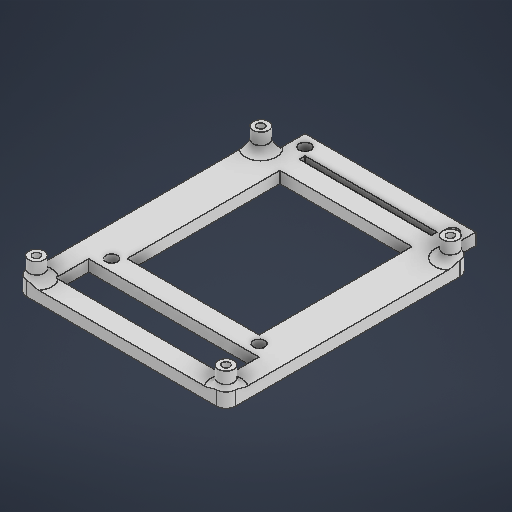
# Autodesk Inventor part: electronics_holder3
Saved by Autodesk Inventor 2026.1 (Build 301233000, 233)
## iProperties
Created: 2026-03-29
Part Number: electronics_holder3
Material: Generic
Document SubType Name: Modeling
Designer: emanuel
Density: 1 g/cm^3
Appearance: Default
Author: emanuel
Autodesk Inventor part; units mm, degrees
ref_plane "YZ Plane" through (0, 0, 0) normal (1, 0, 0) x (0, 1, 0)
ref_plane "XZ Plane" through (0, 0, 0) normal (0, 1, 0) x (-1, 0, 0)
ref_plane "XY Plane" through (0, 0, 0) normal (0, 0, 1) x (1, 0, 0)
sketch "Sketch1" plane through (0, 0, 0) normal (0, 1, 0) x (-1, 0, 0)
  line L0 (-19.075, 25) -> (19.075, 25)
  line L1 (19.075, 25) -> (19.075, -25)
  line L2 (19.075, -25) -> (-19.075, -25)
  line L3 (-19.075, -25) -> (-19.075, 25)
  line L4 (-19.075, 25) -> (19.075, -25) construction
  line L5 (19.075, 25) -> (-19.075, -25) construction
  circle A0 centre (19.075, 25) radius 1.5
  circle A1 centre (19.075, -25) radius 1.5
  circle A2 centre (-19.075, 25) radius 1.5
  circle A3 centre (-19.075, -25) radius 1.5
  line L6 (19.075, 25) -> (22.075, 25)
  line L7 (22.075, 25) -> (22.075, 28)
  line L8 (22.075, 28) -> (19.075, 28)
  line L9 (19.075, 28) -> (19.075, 25)
  line L10 (-19.075, -25) -> (-22.075, -25)
  line L11 (-22.075, -25) -> (-22.075, -28)
  line L12 (-22.075, -28) -> (-19.075, -28)
  line L13 (-19.075, -28) -> (-19.075, -25)
  line L14 (19.075, 25) -> (17.075, 25)
  line L15 (17.075, 25) -> (17.075, 23)
  line L16 (17.075, 23) -> (19.075, 23)
  line L17 (19.075, 23) -> (19.075, 25)
  line L18 (-19.075, -25) -> (-17.075, -25)
  line L19 (-17.075, -25) -> (-17.075, -23)
  line L20 (-17.075, -23) -> (-19.075, -23)
  line L21 (-19.075, -23) -> (-19.075, -25)
  line L22 (17.075, 23) -> (-17.075, 23)
  line L23 (-17.075, 23) -> (-17.075, -23)
  line L24 (-17.075, -23) -> (17.075, -23)
  line L25 (17.075, -23) -> (17.075, 23)
  line L26 (-22.075, -28) -> (22.075, -28)
  line L27 (22.075, -28) -> (22.075, 28)
  line L28 (22.075, 28) -> (-22.075, 28)
  line L29 (-22.075, 28) -> (-22.075, -28)
  point P0 (0, 0)
  dimension "d0" = 38.15
  dimension "d1" = 50
  dimension "d2" = 3
  dimension "d3" = 3
  dimension "d4" = 3
  dimension "d5" = 3
  dimension "d6" = 3
  dimension "d7" = 3
  dimension "d8" = 3
  dimension "d9" = 3
  dimension "d10" = 2
  dimension "d11" = 2
  dimension "d12" = 2
  dimension "d13" = 2
  constraints: 60 end point, 14 parallel, 7 horizontal, 7 perpendicular, 4 centre point, 4 coincident, 2 midpoint
  measures "d0" distance of L1.end L2.end
  measures "d1" distance of L0.end L1.end
  measures "d2" diameter of A0
  measures "d3" diameter of A1
  measures "d4" diameter of A2
  measures "d5" diameter of A3
  measures "d6" distance of L8.end L7.end
  measures "d7" distance of L7.end L6.end
  measures "d8" distance of L12.end L11.end
  measures "d9" distance of L11.end L10.end
  measures "d10" distance of L16.end L15.end
  measures "d11" distance of L15.end L14.end
  measures "d12" distance of L20.end L19.end
  measures "d13" distance of L19.end L18.end
extrude "Extrusion1" add sketch "Sketch1" along normal blind 3 contours A2 L3 A3 L10 L29 L28 L9 A0 L0 | L0 L15 L22 L23 L20 L3 A2 | L0 A0 L1 L16 L15 | L20 L19 L2 A3 L3 | L16 L1 A1 L2 L19 L24 L25 | L9 L8 L7 L6 A0 | A0 L6 L27 L26 L13 A3 L2 A1 L1 | A3 L13 L12 L11 L10
sketch "Sketch2" plane through (0, 3, 0) normal (0, 1, 0) x (1, 0, 0)
  line L0 (0, 0) -> (0, -10)
  line L1 (24.5, -39) -> (-24.5, -39)
  line L2 (-24.5, -39) -> (-24.5, 19)
  line L3 (-24.5, 19) -> (24.5, 19)
  line L4 (24.5, 19) -> (24.5, -39)
  line L5 (24.5, -39) -> (-24.5, 19) construction
  line L6 (-24.5, -39) -> (24.5, 19) construction
  circle A0 centre (-24.5, -39) radius 1
  circle A1 centre (-24.5, 19) radius 1
  circle A2 centre (24.5, -39) radius 1
  circle A3 centre (24.5, 19) radius 1
  line L7 (-24.5, -39) -> (24.5, -39) construction
  line L8 (-24.5, -41.5) -> (24.5, -41.5)
  line L9 (24.5, -36.5) -> (-24.5, -36.5)
  arc A4 (-24.5, -36.5) -> (-24.5, -41.5) centre (-24.5, -39) ccw
  arc A5 (24.5, -41.5) -> (24.5, -36.5) centre (24.5, -39) ccw
  line L10 (24.5, -39) -> (24.5, 19) construction
  line L11 (27, -39) -> (27, 19)
  line L12 (22, 19) -> (22, -39)
  arc A6 (22, -39) -> (27, -39) centre (24.5, -39) ccw
  arc A7 (27, 19) -> (22, 19) centre (24.5, 19) ccw
  line L13 (24.5, 19) -> (-24.5, 19) construction
  line L14 (24.5, 21.5) -> (-24.5, 21.5)
  line L15 (-24.5, 16.5) -> (24.5, 16.5)
  arc A8 (24.5, 16.5) -> (24.5, 21.5) centre (24.5, 19) ccw
  arc A9 (-24.5, 21.5) -> (-24.5, 16.5) centre (-24.5, 19) ccw
  line L16 (-24.5, 19) -> (-24.5, -39) construction
  line L17 (-27, 19) -> (-27, -39)
  line L18 (-22, -39) -> (-22, 19)
  arc A10 (-22, 19) -> (-27, 19) centre (-24.5, 19) ccw
  arc A11 (-27, -39) -> (-22, -39) centre (-24.5, -39) ccw
  point P0 (0, -39)
  point P1 (24.5, -10)
  point P2 (0, 19)
  point P3 (-24.5, -10)
  point P4 (-22, -36.5)
  point P5 (-22, 16.5)
  point P6 (22, 16.5)
  point P7 (22, -36.5)
  dimension "d16" = 10
  dimension "d17" = 49
  dimension "d18" = 58
  dimension "d19" = 2
  dimension "d20" = 2
  dimension "d21" = 2
  dimension "d22" = 2
  dimension "d23" = 5
  dimension "d24" = 5
  dimension "d25" = 5
  dimension "d26" = 5
  constraints: 46 end point, 16 point on circle, 16 tangent, 12 centre point, 7 equal length, 6 midpoint, 4 coincident, 4 perpendicular, 1 horizontal, 1 vertical
  measures "d16" distance of L0.start L0.end
  measures "d17" distance of L2.end L3.end
  measures "d18" distance of L1.end L2.end
  measures "d19" diameter of A0
  measures "d20" diameter of A1
  measures "d21" diameter of A2
  measures "d22" diameter of A3
  measures "d23" diameter of A5
  measures "d24" diameter of A7
  measures "d25" diameter of A9
  measures "d26" diameter of A11
extrude "Extrusion2" add sketch "Sketch2" against normal blind 3 contours A6 L8 A11 L1 | L12 L9 L4 A2 L1 | L1 L18 L9 L12 | L1 A2 L4 A5 A6 | A11 A4 L2 A0 L1 | L1 A0 L2 L9 L18 | L12 L15 L4 L9 | L9 L2 L15 L18 | L4 A8 L11 A5 | L15 L18 L3 L12 | L12 L3 A3 L4 L15 | A4 L17 A9 L2 | L15 L2 A1 L3 L18 | L4 A3 L3 A7 A8 | L3 A10 L14 A7 | A9 A10 L3 A1 L2
sketch "Sketch3" plane through (0, 3, 0) normal (0, 1, 0) x (1, 0, 0)
  circle A0 centre (-24.5, -39) radius 1 projected
  circle A1 centre (-24.5, -39) radius 1
  circle A2 centre (-24.5, -39) radius 2
  circle A3 centre (-24.5, 19) radius 1 projected
  circle A4 centre (-24.5, 19) radius 1
  circle A5 centre (-24.5, 19) radius 2
  circle A6 centre (24.5, 19) radius 1 projected
  circle A7 centre (24.5, 19) radius 1
  circle A8 centre (24.5, 19) radius 2
  circle A9 centre (24.5, -39) radius 1 projected
  circle A10 centre (24.5, -39) radius 1
  circle A11 centre (24.5, -39) radius 2
  point P0 (0, 0)
  dimension "d29" = 2
  dimension "d30" = 4
  dimension "d31" = 2
  dimension "d32" = 4
  dimension "d33" = 2
  dimension "d34" = 4
  dimension "d35" = 2
  dimension "d36" = 4
  constraints: 8 centre point, 8 coincident
  measures "d29" diameter of A1
  measures "d30" diameter of A2
  measures "d31" diameter of A4
  measures "d32" diameter of A5
  measures "d33" diameter of A7
  measures "d34" diameter of A8
  measures "d35" diameter of A10
  measures "d36" diameter of A11
extrude "Extrusion3" add sketch "Sketch3" along normal blind 5
fillet "Fillet1" radius 2 4 edges at (-26.5, 3, -19) (22.5, 3, -19) (22.5, 3, 39) (-26.5, 3, 39)
body "Solid1"
